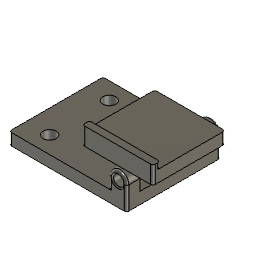
PL Mirror Bracket (Autodesk Fusion 360 design; units mm, degrees)
Autodesk Fusion 360 part; units mm, degrees
sketch "Sketch1" plane through (0, 0, 0) normal (0, 0, 1) x (1, 0, 0) in component "Plate"
  line L0 (25, 20) -> (-25, 20)
  line L1 (-25, 20) -> (-25, -20)
  line L2 (-25, -20) -> (25, -20)
  line L3 (25, -20) -> (25, 20)
  line L4 (25, 20) -> (-25, -20) construction
  line L5 (-25, 20) -> (25, -20) construction
  dimension "d1" = 40
  dimension "d2" = 50
  constraint horizontal L0
  constraint perpendicular L0 L1
  constraint parallel L0 L2
  constraint parallel L1 L3
  constraint coincident L4 origin
  constraint coincident L5 origin
  measures "d1" distance of L0.end L1.end
  measures "d2" distance of L0.start L0.end
extrude "Extrude1" add sketch "Sketch1" along normal blind 5 makes body 1 in component "Plate"
sketch "Sketch2" plane through (0, -20, 0) normal (0, -1, 0) x (1, 0, 0) in component "Plate"
  line L0 (-25, 0) -> (25, 0)
  line L1 (25, 0) -> (25, 5)
  line L2 (25, 5) -> (-25, 5)
  line L3 (-25, 5) -> (-25, 0)
  circle A0 centre (21.25, 9.75) radius 1.75
  circle A1 centre (21.25, 9.75) radius 3.75
  line L4 (25, 9.75) -> (25, 5)
  line L5 (17.5, 9.75) -> (17.5, 5)
  line L6 (21.25, 6) -> (21.25, 5) construction
  dimension "d5" = 3.5
  dimension "d6" = 2
  dimension "d7" = 1
  constraint concentric A0 A1
  constraint coincident A1 L4.start
  constraint tangent A1 L4
  constraint perpendicular L2 L4
  constraint coincident A1 L5.start
  constraint coincident L2 L5.end
  constraint tangent A1 L5
  constraint perpendicular L2 L5
  constraint coincident L1.end L2.start
  constraint coincident A1 L6.start
  constraint coincident L2 L6.end
  constraint perpendicular L2 L6
  constraint vertical A0.centre L6.end
  measures "d5" diameter of A0
  measures "d6" distance of A0 A1
  measures "d7" distance of L6.start L6.end
extrude "Extrude2" add sketch "Sketch2" against normal blind 5.75 contours L2 A1 L4 L5 | A1 bodies 1 in component "Plate"
extrude "Extrude3" add sketch "Sketch2" along normal blind 15 from surface at -40 contours L2 A1 L4 L5 | A1 bodies 1 in component "Plate"
sketch "Sketch1 (2)" plane through (0, 20, 0) normal (0, 1, 0) x (-1, 0, 0) in component "Bolt"
  circle A0 centre (-21.25, 9.75) radius 1.75
  line L0 (-25, 0) -> (25, 0)
  line L1 (25, 0) -> (25, 5)
  line L2 (25, 5) -> (-17.5, 5)
  line L3 (-17.5, 5) -> (-17.5, 9.75)
  arc A1 (-17.5, 9.75) -> (-25, 9.75) centre (-21.25, 9.75) ccw
  line L4 (-25, 9.75) -> (-25, 0)
  circle A2 centre (-21.25, 9.75) radius 2.8
  circle A3 centre (-21.25, 9.75) radius 1.45
  dimension "d13" = 5.6
  dimension "d14" = 2.9
  constraint concentric A0 A2
  constraint concentric A0 A3
  measures "d13" diameter of A2
  measures "d14" diameter of A3
extrude "Extrude1'" add sketch "Sketch1 (2)" against normal blind 27.8 separate body contours A3 makes body 2 in component "Bolt"
extrude "Extrude2'" add sketch "Sketch1 (2)" against normal blind 3 contours A0 | A2 bodies 2 in component "Bolt"
sketch "Sketch3" plane through (0, 20, 0) normal (0, 1, 0) x (-1, 0, 0)
  circle A0 centre (-21.25, 9.75) radius 1.75
  line L0 (-25, 0) -> (25, 0)
  line L1 (25, 0) -> (25, 5)
  line L2 (25, 5) -> (-17.5, 5)
  line L3 (-17.5, 5) -> (-17.5, 9.75)
  arc A1 (-17.5, 9.75) -> (-25, 9.75) centre (-21.25, 9.75) ccw
  line L4 (-25, 9.75) -> (-25, 0)
  circle A2 centre (-21.25, 9.75) radius 3
  dimension "d23" = 6
  constraint concentric A0 A2
  measures "d23" diameter of A2
extrude "Extrude1''" cut sketch "Sketch3" against normal up to surface (13 mm away) contours A2 bodies 1 in component "Plate"
sketch "Sketch4" plane through (0, -20, 0) normal (0, -1, 0) x (1, 0, 0)
  circle A0 centre (21.25, 9.75) radius 1.75
  line L0 (-25, 0) -> (25, 0)
  line L1 (25, 0) -> (25, 9.75)
  arc A1 (25, 9.75) -> (17.5, 9.75) centre (21.25, 9.75) ccw
  line L2 (17.5, 9.75) -> (17.5, 5)
  line L3 (17.5, 5) -> (-25, 5)
  line L4 (-25, 5) -> (-25, 0)
  circle A2 centre (21.25, 9.75) radius 2.25
  dimension "d30" = 4.5
  constraint concentric A0 A2
  measures "d30" diameter of A2
extrude "Extrude2''" cut sketch "Sketch4" against normal blind 5.75 contours A2 bodies 1 in component "Plate"
chamfer "Chamfer1" distance 0.5 angle 45 2 edges at (19.1523, -14.25, 8.9364) (19.1523, -20, 10.5636) on bodies 1 in component "Plate"
extrude "Extrude1'''" add sketch "Sketch2" against normal up to surface (18.85 mm away) from surface at -5.95 separate body contours A1 makes body 3 in component "Mount"
sketch "Sketch5" plane through (0, -14.05, 0) normal (0, -1, 0) x (1, 0, 0)
  circle A0 centre (21.25, 9.75) radius 1.75
  circle A1 centre (21.25, 9.75) radius 3.75
  line L0 (21.25, 13.5) -> (21.25, 15.5) construction
  line L1 (25, 9.75) -> (25, 15.5)
  line L2 (17.5, 9.75) -> (17.5, 15.5)
  line L3 (17.5, 15.5) -> (25, 15.5)
  dimension "d37" = 2
  constraint coincident A1 L0.start
  constraint vertical L0
  constraint vertical A0.centre L0.start
  constraint coincident A1 L1.start
  constraint tangent A1 L1
  constraint vertical L1
  constraint coincident A1 L2.start
  constraint tangent A1 L2
  constraint parallel L1 L2
  constraint equal L1 L2
  constraint horizontal L0.end L1.end
  measures "d37" distance of L0.start L0.end
extrude "Extrude2'''" add sketch "Sketch5" against normal blind 18.85 contours A1 L1 L2 L3 bodies 3 in component "Mount"
sketch "Sketch6" plane through (0, 0, 15.5) normal (0, 0, 1) x (-1, 0, 0)
  line L0 (-17.5, 14.05) -> (-25, 14.05)
  line L1 (-25, 14.05) -> (-25, -4.8)
  line L2 (-25, -4.8) -> (-17.5, -4.8)
  line L3 (-17.5, -4.8) -> (-17.5, 14.05)
  line L4 (25, 20) -> (-17.5, 20)
  line L5 (-17.5, -20) -> (25, -20)
  line L6 (-17.5, -4.8) -> (-25, 14.05) construction
  line L7 (-36.25, -10.75) -> (-6.25, -10.75)
  line L8 (-6.25, -10.75) -> (-6.25, 20)
  line L9 (-6.25, 20) -> (-36.25, 20)
  line L10 (-36.25, 20) -> (-36.25, -10.75)
  line L11 (-36.25, -10.75) -> (-6.25, 20) construction
  line L12 (-6.25, -10.75) -> (-36.25, 20) construction
  point P0 (-21.25, 4.625)
  dimension "d40" = 30
  constraint coincident L2.end L3.start
  constraint coincident L0.end L1.start
  constraint horizontal L7
  constraint perpendicular L7 L8
  constraint parallel L7 L9
  constraint parallel L8 L10
  constraint coincident L11 P0
  constraint coincident L12 P0
  constraint midpoint L6 P0
  constraint collinear L4 L9
  measures "d40" distance of L7.start L7.end
extrude "Extrude3'" add sketch "Sketch6" along normal blind 5 contours L0 L1 L2 L3 | L4 L7 L8 L9 L10 bodies 3 in component "Mount"
sketch "Sketch7" plane through (0, 0, 20.5) normal (0, 0, 1) x (-1, 0, 0)
  line L0 (-36.25, 20) -> (-36.25, -10.75)
  line L1 (-36.25, -10.75) -> (-6.25, -10.75)
  line L2 (-6.25, -10.75) -> (-6.25, 20)
  line L3 (-6.25, 20) -> (-36.25, 20)
  line L4 (-6.25, 20) -> (-36.25, 20)
  line L5 (-36.25, 20) -> (-36.25, 17)
  line L6 (-36.25, 17) -> (-6.25, 17)
  line L7 (-6.25, 17) -> (-6.25, 20)
  dimension "d43" = 3
  constraint horizontal L4
  constraint vertical L5
  constraint horizontal L6
  constraint vertical L7
  constraint coincident L0 L5.end
  constraint coincident L2.end L3.start
  measures "d43" distance of L2.end L6.end
extrude "Extrude4" add sketch "Sketch7" along normal blind 2.5 contours L0 L2 L3 L4 L5 L6 L7 bodies 3 in component "Mount"
fillet "Fillet1" radius 1 4 edges at (6.25, 10.75, 18) (6.25, -20, 19.25) (36.25, 10.75, 18) (36.25, -20, 19.25) on bodies 3 in component "Mount"
fillet "Fillet1'" radius 1 8 edges at (-25, 20, 2.5) (-25, -20, 2.5) (25, 20, 4.875) (21.25, 20, 13.5) (17.5, 20, 7.375) (25, -20, 4.875) (21.25, -20, 13.5) (17.5, -20, 7.375) on bodies 1 in component "Plate"
fillet "Fillet2" radius 1 2 edges at (36.25, -17, 21.75) (6.25, -17, 21.75) on bodies 3 in component "Mount"
sketch "Sketch8" plane through (0, 0, 5) normal (0, 0, 1) x (-1, 0, 0)
  arc A0 (25, 19) -> (24, 20) centre (24, 19) ccw
  line L0 (24, 20) -> (-18.5, 20)
  arc A1 (-17.5, 19) -> (-18.5, 20) centre (-18.5, 19) ccw
  line L1 (-17.5, 19) -> (-17.5, 14.25)
  line L2 (-17.5, 14.25) -> (-25, 14.25)
  line L3 (-25, 14.25) -> (-25, -5)
  line L4 (-25, -5) -> (-17.5, -5)
  line L5 (-17.5, -5) -> (-17.5, -19)
  arc A2 (-18.5, -20) -> (-17.5, -19) centre (-18.5, -19) ccw
  line L6 (-18.5, -20) -> (24, -20)
  arc A3 (24, -20) -> (25, -19) centre (24, -19) ccw
  line L7 (25, -19) -> (25, 19)
  line L8 (25, 0) -> (15, 0) construction
  circle A4 centre (15, -12.7) radius 2.75
  circle A5 centre (15, 12.7) radius 2.75
  dimension "d52" = 12.7
  dimension "d53" = 5.5
  dimension "d54" = 10
  constraint midpoint L7 L8.start
  constraint perpendicular L7 L8
  constraint vertical L8.end A4.centre
  constraint symmetric L8 A4 A5
  measures "d52" distance of L8 A4.centre
  measures "d53" diameter of A4
  measures "d54" distance of L8.start L8.end
extrude "Extrude3''" cut sketch "Sketch8" against normal blind 5 contours A4 | A5 bodies 1 in component "Plate"
component "Bolt" placed x (1, 0, 0) y (0, 1, 0) z (0, 0, 1) at (0, -10, 0)
component "Plate" placed x (1, 0, 0) y (0, 1, 0) z (0, 0, 1) at (0, 0, 0)
component "Mount" placed x (1, 0, 0) y (0, 1, 0) z (0, 0, 1) at (0, 0, 0)
equation "d52 = 1 in / 2"
